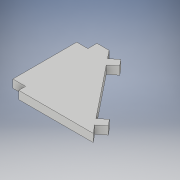
# Autodesk Inventor part: Part Siku
Saved by Autodesk Inventor 2019 (Build 230136000, 136)
## iProperties
Created: 2019-07-09
Part Number: Part Siku
Material: Generic
Document SubType Name: Modeling
Designer: azriel
Density: 1 g/cm^3
Appearance: Default
Author: azriel
Autodesk Inventor part; units mm, degrees
ref_plane "YZ Plane" through (0, 0, 0) normal (1, 0, 0) x (0, 1, 0)
ref_plane "XZ Plane" through (0, 0, 0) normal (0, 1, 0) x (-1, 0, 0)
ref_plane "XY Plane" through (0, 0, 0) normal (0, 0, 1) x (1, 0, 0)
sketch "Sketch1" plane through (0, 0, 0) normal (0, 1, 0) x (-1, 0, 0)
  line L0 (35.9534, 25.7381) -> (34.9534, 25.7381)
  line L1 (28.381, 30.0256) -> (-11.619, 30.0256)
  line L2 (-11.619, 30.0256) -> (28.381, -19.9744)
  line L3 (-7.619, 25.0256) -> (-12.3042, 21.2774)
  line L4 (-12.3042, 21.2774) -> (-9.1808, 17.3731)
  line L5 (-9.1808, 17.3731) -> (-4.4956, 21.1213)
  line L6 (24.381, -14.9744) -> (19.6958, -18.7226)
  line L7 (19.6958, -18.7226) -> (16.5723, -14.8182)
  line L8 (16.5723, -14.8182) -> (21.2575, -11.0701)
  line L9 (30.9534, 30.0256) -> (28.381, 30.0256)
  line L10 (34.9534, 25.7381) -> (38.9534, 25.7381)
  line L11 (35.9534, -14.2619) -> (42.9534, -14.2619)
  line L12 (30.9534, -19.9744) -> (28.381, -19.9744)
  line L13 (30.9534, -19.9744) -> (35.9534, -19.9744)
  line L14 (35.9534, -19.9744) -> (35.9534, -14.2619)
  line L15 (35.9534, -14.2619) -> (42.9534, -14.2619)
  line L16 (42.9534, -14.2619) -> (42.9534, 25.7381)
  line L17 (42.9534, 25.7381) -> (38.9534, 25.7381)
  line L18 (30.9534, 30.0256) -> (34.9534, 30.0256)
  line L19 (34.9534, 30.0256) -> (34.9534, 25.7381)
  point P0 (0, 0)
  dimension "d4" = 40
  dimension "d5" = 6
  dimension "d6" = 5
  dimension "d9" = 5
  dimension "d10" = 6
  dimension "d18" = 7
  constraints: 40 end point, 6 perpendicular, 5 point on line, 3 horizontal, 1 collinear
  measures "d4" distance of L1.start L1.end
  measures "d5" distance of L3.start L3.end
  measures "d6" distance of L3.end L4.end
  measures "d9" distance of L6.end L7.end
  measures "d10" distance of L7.end L8.end
  measures "d18" distance of L11.end L11.start
extrude "Extrusion1" add sketch "Sketch1" along normal blind 5
body "Solid1"
